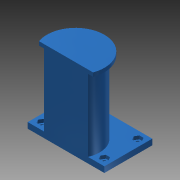
# Autodesk Inventor part: SpoolHolderSingle
Saved by Autodesk Inventor 2015 SP1 (Build 190203100, 203)
## iProperties
Created: 2015-04-19
Part Number: SpoolHolderSingle
Material: ABS Plastic
Document SubType Name: Modeling
Designer: Jack
Density: 1.06 g/cm^3
Appearance: Cyan
Author: Jack
Autodesk Inventor part; units mm, degrees
ref_plane "YZ Plane" through (0, 0, 0) normal (1, 0, 0) x (0, 1, 0)
ref_plane "XZ Plane" through (0, 0, 0) normal (0, 1, 0) x (-1, 0, 0)
ref_plane "XY Plane" through (0, 0, 0) normal (0, 0, 1) x (1, 0, 0)
sketch "Sketch1" plane through (0, 0, 0) normal (0, 0, 1) x (1, 0, 0)
  line L0 (0, 0) -> (80, 0)
  line L1 (80, 0) -> (80, 50)
  line L2 (80, 50) -> (0, 50)
  line L3 (0, 50) -> (0, 0)
  dimension "d0" = 80
  dimension "d1" = 50
  constraints: 8 end point, 2 parallel, 1 horizontal, 1 perpendicular
  measures "d0" distance of L2.end L1.end
  measures "d1" distance of L1.end L0.end
extrude "Extrusion1" add sketch "Sketch1" along normal blind 6
sketch "Sketch2" plane through (0, 0, 6) normal (0, 0, 1) x (1, 0, 0)
  line L0 (80, 50) -> (0, 50) projected
  line L1 (0, 50) -> (0, 0) projected
  arc A0 (62.9129, 0) -> (17.0871, 0) centre (40, 10) ccw
  line L2 (17.0871, 0) -> (62.9129, 0)
  dimension "d11" = 50
  dimension "d12" = 40
  dimension "d13" = 40
  dimension "d14" = 10
  constraints: 2 end point, 2 point on circle, 1 centre point, 1 horizontal
  measures "d11" diameter of A0
  measures "d12" distance from line of L0 A0.centre
  measures "d13" distance from line of L1 A0.centre
  measures "d14" distance from line of A0.centre L2
extrude "Extrusion2" add sketch "Sketch2" along normal blind 75
sketch "Sketch8" plane through (0, 0, 81) normal (0, 0, 1) x (1, 0, 0)
  arc A0 (62.9129, 0) -> (17.0871, 0) centre (40, 10) ccw projected
  line L0 (17.0871, 0) -> (62.9129, 0) projected
  arc A1 (68.2843, 0) -> (11.7157, 0) centre (40, 10) ccw
  line L1 (17.0871, 0) -> (11.7157, 0)
  line L2 (62.9129, 0) -> (68.2843, 0)
  point P0 (0, 0)
  dimension "d30" = 60
  constraints: 4 end point, 2 point on circle, 1 centre point, 1 coincident, 1 horizontal, 1 point on line
  measures "d30" diameter of A1
extrude "Extrusion7" add sketch "Sketch8" along normal blind 4
sketch "Sketch9" plane through (0, 0, 0) normal (0, 0, -1) x (-1, 0, 0)
  line L0 (0, 0) -> (-80, 0) projected
  line L1 (-80, 0) -> (-80, 50) projected
  point P0 (-72.5, 42.5)
  point P1 (-72.5, 7.5)
  point P2 (-7.5, 42.5)
  point P3 (-7.5, 7.5)
  dimension "d33" = 65
  dimension "d34" = 35
  dimension "d35" = 7.5
  dimension "d36" = 7.5
  constraints: 2 horizontal alignment, 2 vertical alignment
  measures "d33" distance of point (-7.5, 42.5) point (-72.5, 42.5)
  measures "d34" distance of point (-72.5, 42.5) point (-72.5, 7.5)
  measures "d35" distance from line of L1 point (-72.5, 42.5)
  measures "d36" distance from line of point (-72.5, 7.5) L0
hole "Hole1" at (72.5, 42.5, 0) at (72.5, 7.5, 0) at (7.5, 42.5, 0) at (7.5, 7.5, 0) direction (0, 0, 1) diameter 4.5 end through all
sketch "Sketch10" plane through (0, 0, 6) normal (0, 0, 1) x (1, 0, 0)
  circle A0 centre (7.5, 42.5) radius 2.25 projected
  circle A1 centre (72.5, 42.5) radius 2.25 projected
  circle A2 centre (72.5, 7.5) radius 2.25 projected
  circle A3 centre (7.5, 7.5) radius 2.25 projected
  line L0 (11.7724, 42.5) -> (9.6362, 38.8)
  line L1 (9.6362, 38.8) -> (5.3638, 38.8)
  line L2 (5.3638, 38.8) -> (3.2276, 42.5)
  line L3 (3.2276, 42.5) -> (5.3638, 46.2)
  line L4 (5.3638, 46.2) -> (9.6362, 46.2)
  line L5 (9.6362, 46.2) -> (11.7724, 42.5)
  line L6 (11.7724, 7.5) -> (9.6362, 3.8)
  line L7 (9.6362, 3.8) -> (5.3638, 3.8)
  line L8 (5.3638, 3.8) -> (3.2276, 7.5)
  line L9 (3.2276, 7.5) -> (5.3638, 11.2)
  line L10 (5.3638, 11.2) -> (9.6362, 11.2)
  line L11 (9.6362, 11.2) -> (11.7724, 7.5)
  line L12 (76.7724, 7.5) -> (74.6362, 3.8)
  line L13 (74.6362, 3.8) -> (70.3638, 3.8)
  line L14 (70.3638, 3.8) -> (68.2276, 7.5)
  line L15 (68.2276, 7.5) -> (70.3638, 11.2)
  line L16 (70.3638, 11.2) -> (74.6362, 11.2)
  line L17 (74.6362, 11.2) -> (76.7724, 7.5)
  line L18 (76.7724, 42.5) -> (74.6362, 38.8)
  line L19 (74.6362, 38.8) -> (70.3638, 38.8)
  line L20 (70.3638, 38.8) -> (68.2276, 42.5)
  line L21 (68.2276, 42.5) -> (70.3638, 46.2)
  line L22 (70.3638, 46.2) -> (74.6362, 46.2)
  line L23 (74.6362, 46.2) -> (76.7724, 42.5)
  dimension "d44" = 7.4
  constraints: 48 end point, 4 coincident, 4 horizontal, 3 equal length, 52 other
  measures "d44" distance between parallel lines of L7 L10
extrude "Extrusion8" cut sketch "Sketch10" against normal blind 3.5
sketch "Sketch4" plane through (0, 0, 26) normal (0, 0, 1) x (1, 0, 0)
  arc A0 (62.9129, 0) -> (17.0871, 0) centre (40, 10) ccw projected
  line L0 (17.0871, 0) -> (62.9129, 0) projected
  circle A1 centre (40, 24.5) radius 11 construction
  arc A2 (28, 24.5) -> (52, 24.5) centre (40, 24.5) ccw
  line L1 (28, 24.5) -> (28, 31.9317)
  line L2 (52, 24.5) -> (52, 31.9317)
  arc A3 (62.9129, 0) -> (17.0871, 0) centre (40, 10) ccw projected
  point P0 (0, 0)
  dimension "d15" = 22
  dimension "d16" = 14.5
  dimension "d17" = 24
  constraints: 5 point on circle, 4 end point, 2 centre point, 2 tangent, 2 vertical, 1 coincident, 1 vertical alignment
  measures "d15" diameter of A1
  measures "d16" distance of A0.centre A1.centre
  measures "d17" diameter of A2
sketch "Sketch5" plane through (0, 0, 61) normal (0, 0, 1) x (1, 0, 0)
  arc A0 (62.9129, 0) -> (17.0871, 0) centre (40, 10) ccw projected
  line L0 (17.0871, 0) -> (62.9129, 0) projected
  arc A1 (28, 24.5) -> (52, 24.5) centre (40, 24.5) ccw projected
  line L1 (52, 31.9317) -> (52, 24.5) projected
  arc A2 (52, 31.9317) -> (28, 31.9317) centre (40, 10) ccw projected
  line L2 (28, 24.5) -> (28, 31.9317) projected
  point P0 (0, 0)
sketch "Sketch6" plane through (0, 0, 26) normal (0, 0, 1) x (1, 0, 0)
  arc A0 (28, 24.5) -> (52, 24.5) centre (40, 24.5) ccw projected
  line L0 (52, 31.9317) -> (52, 24.5) projected
  arc A1 (52, 31.9317) -> (28, 31.9317) centre (40, 10) ccw projected
  line L1 (28, 24.5) -> (28, 31.9317) projected
  arc A2 (35.75, 24.5) -> (44.25, 24.5) centre (40, 24.5) ccw
  line L2 (35.75, 26.9) -> (35.75, 34.6361)
  arc A3 (52, 31.9317) -> (28, 31.9317) centre (40, 10) ccw projected
  line L3 (44.25, 26.9) -> (44.25, 34.6361)
  arc A4 (35.75, 24.5) -> (35.75, 26.9) centre (34.15, 25.7) ccw
  arc A5 (44.25, 26.9) -> (44.25, 24.5) centre (45.85, 25.7) ccw
  point P0 (0, 0)
  dimension "d23" = 8.5
  dimension "d24" = 2
  dimension "d25" = 1.6
  constraints: 10 point on circle, 4 end point, 3 centre point, 2 tangent, 2 vertical, 2 vertical alignment, 1 coincident, 1 equal radius, 1 horizontal alignment
  measures "d23" diameter of A2
  measures "d24" radius of A4
  measures "d25" distance from line of L2 A4.centre
sketch "Sketch7" plane through (0, 0, 61) normal (0, 0, 1) x (1, 0, 0)
  arc A0 (35.75, 24.5) -> (44.25, 24.5) centre (40, 24.5) ccw projected
  arc A1 (44.25, 26.9) -> (44.25, 24.5) centre (45.85, 25.7) ccw projected
  line L0 (44.25, 34.6361) -> (44.25, 26.9) projected
  arc A2 (44.25, 34.6361) -> (35.75, 34.6361) centre (40, 10) ccw projected
  line L1 (35.75, 26.9) -> (35.75, 34.6361) projected
  arc A3 (35.75, 24.5) -> (35.75, 26.9) centre (34.15, 25.7) ccw projected
  point P0 (0, 0)
body "Solid1"
